Autodesk Fusion 360 part; units mm, degrees
(part 2 of 2)
  measures "d118" distance of L392.end L396.end
  measures "d119" distance of L392.end L398.end
  measures "d120" distance of L397.end L400.end
  measures "d121" distance of L397.end L402.end
  measures "d122" distance of L360.end L408.end
  measures "d123" distance of L360.end L410.end
  measures "d124" distance of L409.end L412.end
  measures "d125" distance of L409.end L414.end
  measures "d126" distance of L376.end L416.end
  measures "d127" distance of L376.end L418.end
  measures "d128" distance of L417.end L420.end
  measures "d129" distance of L417.end L422.end
  measures "d130" distance of L421.end L424.end
  measures "d131" distance of L421.end L426.end
  measures "d132" distance of L425.end L434.end
  measures "d133" distance of L420.end L436.end
  measures "d134" distance of L420.end L438.end
  measures "d135" distance of L437.end L442.end
  measures "d136" distance of L442.end L444.end
  measures "d137" distance of L442.end L446.end
  measures "d138" distance of L446.end L452.end
  measures "d139" distance of L446.end L454.end
  measures "d140" distance of L436.end L424.end
extrude "Extrude11" add sketch "Sketch9" along normal blind 67 separate body contours L336 L339 L340 L341 L342 L343 | L241 L242 L245 L246 L299 L300 L307 L308 L328 L329 L330 L331 L333 L334 | L333 L334 L480 | L336 L341 L388 L407 | L339 L342 L386 L391 | L336 L398 L404 L405 L406 L407 | L388 L389 L390 L391 | L339 L384 L385 L386 L387 | L336 L398 L403 L405 | L389 L392 L399 L404 | L382 L387 L390 L395 | L339 L381 L384 L468 | L336 L400 L401 L402 L403 | L396 L397 L398 L399 L404 | L392 L393 L394 L395 | L380 L381 L382 L383 | L339 L468 L469 L470 L471 | L336 L337 L345 L346 L397 L400 L401 L446 L450 L451 L454 L455 | L377 L378 L383 L393 L394 L396 L416 L445 L448 L449 L456 L457 | L374 L379 L380 L471 | L339 L370 L375 L470 | L336 L337 L344 L345 L346 L347 | L448 L449 L450 L451 | L376 L377 L378 L379 | L372 L373 L374 L375 | L339 L368 L369 L370 L371 | L373 L376 L419 L474 | L366 L371 L372 L475 | L339 L365 L368 L466 | L444 L445 L446 L447 | L416 L417 L418 L419 | L472 L473 L474 L475 | L364 L365 L366 L367 | L339 L464 L465 L466 L467 | L337 L452 L453 L454 L455 | L438 L443 L444 L459 | L456 L457 L458 L459 | L337 L442 L447 L452 | L417 L420 L439 L458 | L361 L362 L367 L408 L418 L422 L423 L427 L428 L429 L472 L473 | L358 L363 L364 L467 | L339 L354 L359 L464 | L337 L440 L441 L442 L443 | L436 L437 L438 L439 | L420 L421 L422 L423 | L360 L361 L362 L363 | L356 L357 L358 L359 | L338 L339 L352 L353 L354 L355 | L337 L437 L440 L460 | L421 L424 L436 L463 | L357 L360 L411 L476 | L338 L353 L356 L479 | L337 L460 L461 L462 L463 | L424 L425 L426 L427 | L408 L409 L410 L411 | L338 L476 L477 L478 L479 | L337 L425 L432 L462 | L337 L338 L349 L350 L409 L412 L413 L426 L430 L431 L434 L435 | L428 L429 L430 L431 | L338 L410 L415 L477 | L337 L432 L433 L434 L435 | L338 L412 L413 L414 L415 | L337 L338 L348 L349 L350 L351 makes body 37
extrude "Extrude12" cut sketch "Sketch9" along normal blind 67 and the other way blind -3 contours L336 L339 L340 L341 L342 L343 | L336 L398 L404 L405 L406 L407 | L339 L384 L385 L386 L387 | L336 L400 L401 L402 L403 | L392 L393 L394 L395 | L339 L468 L469 L470 L471 | L336 L337 L344 L345 L346 L347 | L448 L449 L450 L451 | L376 L377 L378 L379 | L339 L368 L369 L370 L371 | L472 L473 L474 L475 | L339 L464 L465 L466 L467 | L337 L452 L453 L454 L455 | L456 L457 L458 L459 | L337 L440 L441 L442 L443 | L420 L421 L422 L423 | L360 L361 L362 L363 | L338 L339 L352 L353 L354 L355 | L337 L460 L461 L462 L463 | L338 L476 L477 L478 L479 | L428 L429 L430 L431 | L337 L432 L433 L434 L435 | L338 L412 L413 L414 L415 | L337 L338 L348 L349 L350 L351 bodies 37
copy_body "CopyPasteBodies35" bodies 37 makes body 38
move_body "Move52" bodies 38 to x (1, 0, 0) y (0, 1, 0) z (0, 0, 1) at (-99, 0, -141)
copy_body "CopyPasteBodies36" bodies 38 makes body 39
move_body "Move53" bodies 39 to x (1, 0, 0) y (0, 1, 0) z (0, 0, 1) at (-99, 0, 0)
hidden bodies 1 36 37 38
equation "d1 = ( 14 * 3 ) * 1 mm"
equation "d4 = ( 14 * 3 ) * 1 mm"
equation "d5 = ( 14 * 5 ) * 1 mm"
equation "d8 = ( 14 * 3 ) * 1 mm"
equation "d10 = ( 14 * 3 ) * 1 mm"
equation "d11 = ( 14 * 3 ) * 1 mm"
equation "d14 = ( 14 * 3 ) * 1 mm"
equation "d15 = ( 14 * 3 ) * 1 mm"
equation "d18 = ( 14 * 3 ) * 1 mm"
equation "d26 = 42.000 mm + 7 mm"
equation "d88 = ( 18.2 * 4 ) * 1 mm + 1 mm"
equation "d89 = ( 18.2 * 6 ) * 1 mm + 2 mm"
